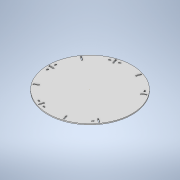
# Autodesk Inventor part: Base
Saved by Autodesk Inventor 2020 (Build 240168000, 168)
## iProperties
Created: 2020-07-30
Part Number: Base
Material: Generic
Document SubType Name: Modeling
Designer: Dan Wikman
Density: 1 g/cm^3
Appearance: Default
Author: Dan Wikman
Autodesk Inventor part; units mm, degrees
ref_plane "YZ Plane" through (0, 0, 0) normal (1, 0, 0) x (0, 1, 0)
ref_plane "XZ Plane" through (0, 0, 0) normal (0, 1, 0) x (-1, 0, 0)
ref_plane "XY Plane" through (0, 0, 0) normal (0, 0, 1) x (1, 0, 0)
sketch "Sketch1" plane through (0, 0, 0) normal (0, 1, 0) x (-1, 0, 0)
  circle A0 centre (0, 0) radius 300
  line L0 (290, 3.75) -> (260, 3.75)
  line L1 (260, -3.75) -> (290, -3.75)
  arc A1 (291.75, 2) -> (290, 3.75) centre (290, 2) ccw
  arc A2 (290, -3.75) -> (291.75, -2) centre (290, -2) ccw
  arc A3 (258.25, -2) -> (260, -3.75) centre (260, -2) ccw
  arc A4 (260, 3.75) -> (258.25, 2) centre (260, 2) ccw
  line L2 (258.25, 2) -> (258.25, -2)
  line L3 (291.75, -2) -> (291.75, 2)
  line L4 (306.241, 0) -> (300, 0)
  line L5 (300, 0) -> (281.7438, 0)
  line L6 (232.4107, 173.4915) -> (208.1402, 155.858)
  arc A5 (234.8551, 173.1044) -> (232.4107, 173.4915) centre (233.4394, 172.0758) ccw
  line L7 (237.2063, 169.8683) -> (234.8551, 173.1044)
  line L8 (212.5486, 149.7904) -> (236.8191, 167.4239)
  arc A6 (236.8191, 167.4239) -> (237.2063, 169.8683) centre (235.7905, 168.8397) ccw
  arc A7 (208.1402, 155.858) -> (207.7531, 153.4136) centre (209.1688, 154.4422) ccw
  line L9 (207.7531, 153.4136) -> (210.1042, 150.1775)
  arc A8 (210.1042, 150.1775) -> (212.5486, 149.7904) centre (211.52, 151.2061) ccw
  line L10 (86.0485, 276.9652) -> (76.778, 248.4335)
  arc A9 (88.2536, 278.0888) -> (86.0485, 276.9652) centre (87.7128, 276.4244) ccw
  line L11 (92.0578, 276.8527) -> (88.2536, 278.0888)
  line L12 (83.9109, 246.1159) -> (93.1814, 274.6476)
  arc A10 (93.1814, 274.6476) -> (92.0578, 276.8527) centre (91.517, 275.1884) ccw
  arc A11 (76.778, 248.4335) -> (77.9015, 246.2284) centre (78.4423, 247.8927) ccw
  line L13 (77.9015, 246.2284) -> (81.7058, 244.9923)
  arc A12 (81.7058, 244.9923) -> (83.9109, 246.1159) centre (82.2465, 246.6567) ccw
  line L14 (-93.1814, 274.6476) -> (-83.9109, 246.1159)
  arc A13 (-92.0578, 276.8527) -> (-93.1814, 274.6476) centre (-91.517, 275.1884) ccw
  line L15 (-88.2536, 278.0888) -> (-92.0578, 276.8527)
  line L16 (-76.778, 248.4335) -> (-86.0485, 276.9652)
  arc A14 (-86.0485, 276.9652) -> (-88.2536, 278.0888) centre (-87.7128, 276.4244) ccw
  arc A15 (-83.9109, 246.1159) -> (-81.7058, 244.9923) centre (-82.2465, 246.6567) ccw
  line L17 (-81.7058, 244.9923) -> (-77.9015, 246.2284)
  arc A16 (-77.9015, 246.2284) -> (-76.778, 248.4335) centre (-78.4423, 247.8927) ccw
  line L18 (-236.8191, 167.4239) -> (-212.5486, 149.7904)
  arc A17 (-237.2063, 169.8683) -> (-236.8191, 167.4239) centre (-235.7905, 168.8397) ccw
  line L19 (-234.8551, 173.1044) -> (-237.2063, 169.8683)
  line L20 (-208.1402, 155.858) -> (-232.4107, 173.4915)
  arc A18 (-232.4107, 173.4915) -> (-234.8551, 173.1044) centre (-233.4394, 172.0758) ccw
  arc A19 (-212.5486, 149.7904) -> (-210.1042, 150.1775) centre (-211.52, 151.2061) ccw
  line L21 (-210.1042, 150.1775) -> (-207.7531, 153.4136)
  arc A20 (-207.7531, 153.4136) -> (-208.1402, 155.858) centre (-209.1688, 154.4422) ccw
  line L22 (-232.4107, -173.4915) -> (-208.1402, -155.858)
  arc A21 (-234.8551, -173.1044) -> (-232.4107, -173.4915) centre (-233.4394, -172.0758) ccw
  line L23 (-237.2063, -169.8683) -> (-234.8551, -173.1044)
  line L24 (-212.5486, -149.7904) -> (-236.8191, -167.4239)
  arc A22 (-236.8191, -167.4239) -> (-237.2063, -169.8683) centre (-235.7905, -168.8397) ccw
  arc A23 (-208.1402, -155.858) -> (-207.7531, -153.4136) centre (-209.1688, -154.4422) ccw
  line L25 (-207.7531, -153.4136) -> (-210.1042, -150.1775)
  arc A24 (-210.1042, -150.1775) -> (-212.5486, -149.7904) centre (-211.52, -151.2061) ccw
  line L26 (-86.0485, -276.9652) -> (-76.778, -248.4335)
  arc A25 (-88.2536, -278.0888) -> (-86.0485, -276.9652) centre (-87.7128, -276.4244) ccw
  line L27 (-92.0578, -276.8527) -> (-88.2536, -278.0888)
  line L28 (-83.9109, -246.1159) -> (-93.1814, -274.6476)
  arc A26 (-93.1814, -274.6476) -> (-92.0578, -276.8527) centre (-91.517, -275.1884) ccw
  arc A27 (-76.778, -248.4335) -> (-77.9015, -246.2284) centre (-78.4423, -247.8927) ccw
  line L29 (-77.9015, -246.2284) -> (-81.7058, -244.9923)
  arc A28 (-81.7058, -244.9923) -> (-83.9109, -246.1159) centre (-82.2465, -246.6567) ccw
  line L30 (93.1814, -274.6476) -> (83.9109, -246.1159)
  arc A29 (92.0578, -276.8527) -> (93.1814, -274.6476) centre (91.517, -275.1884) ccw
  line L31 (88.2536, -278.0888) -> (92.0578, -276.8527)
  line L32 (76.778, -248.4335) -> (86.0485, -276.9652)
  arc A30 (86.0485, -276.9652) -> (88.2536, -278.0888) centre (87.7128, -276.4244) ccw
  arc A31 (83.9109, -246.1159) -> (81.7058, -244.9923) centre (82.2465, -246.6567) ccw
  line L33 (81.7058, -244.9923) -> (77.9015, -246.2284)
  arc A32 (77.9015, -246.2284) -> (76.778, -248.4335) centre (78.4423, -247.8927) ccw
  line L34 (236.8191, -167.4239) -> (212.5486, -149.7904)
  arc A33 (237.2063, -169.8683) -> (236.8191, -167.4239) centre (235.7905, -168.8397) ccw
  line L35 (234.8551, -173.1044) -> (237.2063, -169.8683)
  line L36 (208.1402, -155.858) -> (232.4107, -173.4915)
  arc A34 (232.4107, -173.4915) -> (234.8551, -173.1044) centre (233.4394, -172.0758) ccw
  arc A35 (212.5486, -149.7904) -> (210.1042, -150.1775) centre (211.52, -151.2061) ccw
  line L37 (210.1042, -150.1775) -> (207.7531, -153.4136)
  arc A36 (207.7531, -153.4136) -> (208.1402, -155.858) centre (209.1688, -154.4422) ccw
  point P0 (227.9355, 165.6049)
  point P1 (87.0636, 267.9543)
  point P2 (-87.0636, 267.9543)
  point P3 (-227.9355, 165.6049)
  point P4 (-227.9355, -165.6049)
  point P5 (-87.0636, -267.9543)
  point P6 (87.0636, -267.9543)
  point P7 (227.9355, -165.6049)
  dimension "d36" = 600
  dimension "d3" = 7.5
  dimension "d6" = 30
  dimension "d7" = 3.5
  dimension "d8" = 3.5
  dimension "d26" = 8.25
  dimension "d27" = 33.5
  dimension "d28" = 7.5
  constraints: 76 end point, 72 point on circle, 36 centre point, 4 tangent, 3 horizontal, 1 horizontal alignment, 1 parallel, 3 other
  measures "d3" distance between parallel lines of L1 L0
  measures "d6" distance of L1.start L1.end
  measures "d7" diameter of A1
  measures "d8" diameter of A2
  measures "d26" distance from line of L4.end L3
  measures "d27" distance between parallel lines of L2 L3
  measures "d28" diameter of L1 L5
extrude "Extrusion1" add sketch "Sketch1" along normal blind 7
sketch "Sketch2" plane through (0, 7, 0) normal (0, 1, 0) x (1, 0, 0)
  circle A0 centre (0, 0) radius 300 projected
  arc A1 (-260, -3.75) -> (-258.25, -2) centre (-260, -2) ccw projected
  line L0 (-260, -3.75) -> (-290, -3.75) projected
  arc A2 (-291.75, -2) -> (-290, -3.75) centre (-290, -2) ccw projected
  line L1 (-291.75, -2) -> (-291.75, 2) projected
  arc A3 (-290, 3.75) -> (-291.75, 2) centre (-290, 2) ccw projected
  line L2 (-290, 3.75) -> (-260, 3.75) projected
  arc A4 (-258.25, 2) -> (-260, 3.75) centre (-260, 2) ccw projected
  line L3 (-258.25, 2) -> (-258.25, -2) projected
  line L4 (-277, 22) -> (-273, 22)
  line L5 (-271.25, 23.75) -> (-271.25, 33.75)
  line L6 (-273, 35.5) -> (-277, 35.5)
  line L7 (-278.75, 33.75) -> (-278.75, 23.75)
  arc A5 (-273, 22) -> (-271.25, 23.75) centre (-273, 23.75) ccw
  arc A6 (-278.75, 23.75) -> (-277, 22) centre (-277, 23.75) ccw
  arc A7 (-277, 35.5) -> (-278.75, 33.75) centre (-277, 33.75) ccw
  arc A8 (-271.25, 33.75) -> (-273, 35.5) centre (-273, 33.75) ccw
  line L8 (-300, 0) -> (0, 0)
  line L9 (-277, -22) -> (-273, -22)
  line L10 (-271.25, -23.75) -> (-271.25, -33.75)
  line L11 (-273, -35.5) -> (-277, -35.5)
  line L12 (-278.75, -33.75) -> (-278.75, -23.75)
  arc A9 (-271.25, -23.75) -> (-273, -22) centre (-273, -23.75) ccw
  arc A10 (-277, -22) -> (-278.75, -23.75) centre (-277, -23.75) ccw
  arc A11 (-278.75, -33.75) -> (-277, -35.5) centre (-277, -33.75) ccw
  arc A12 (-273, -35.5) -> (-271.25, -33.75) centre (-273, -33.75) ccw
  arc A13 (-105.2849, -252.8401) -> (-106.4085, -250.6349) centre (-106.9492, -252.2993) ccw
  arc A14 (-119.3602, -252.4726) -> (-118.2366, -254.6777) centre (-117.6959, -253.0133) ccw
  line L13 (-118.1241, -248.6683) -> (-119.3602, -252.4726)
  arc A15 (-115.919, -247.5448) -> (-118.1241, -248.6683) centre (-116.4598, -249.2091) ccw
  line L14 (-106.4085, -250.6349) -> (-115.919, -247.5448)
  line L15 (-106.521, -256.6443) -> (-105.2849, -252.8401)
  arc A16 (-108.7261, -257.7679) -> (-106.521, -256.6443) centre (-108.1853, -256.1035) ccw
  line L16 (-118.2366, -254.6777) -> (-108.7261, -257.7679)
  line L17 (-64.6745, -270.241) -> (-63.4384, -266.4368)
  arc A17 (-61.2333, -265.3132) -> (-63.4384, -266.4368) centre (-61.774, -266.9776) ccw
  arc A18 (-64.6745, -270.241) -> (-63.5509, -272.4462) centre (-63.0101, -270.7818) ccw
  line L18 (-61.2333, -265.3132) -> (-51.7227, -268.4034)
  line L19 (-54.0403, -275.5363) -> (-63.5509, -272.4462)
  arc A19 (-50.5991, -270.6085) -> (-51.7227, -268.4034) centre (-52.2635, -270.0678) ccw
  line L20 (-50.5991, -270.6085) -> (-51.8352, -274.4128)
  arc A20 (-54.0403, -275.5363) -> (-51.8352, -274.4128) centre (-53.4996, -273.872) ccw
  arc A21 (207.9304, -178.2637) -> (205.486, -178.6509) centre (206.9017, -179.6795) ccw
  arc A22 (203.2313, -191.5366) -> (205.6757, -191.1495) centre (204.26, -190.1208) ccw
  line L21 (199.9953, -189.1855) -> (203.2313, -191.5366)
  arc A23 (199.6081, -186.7411) -> (199.9953, -189.1855) centre (201.0239, -187.7697) ccw
  line L22 (205.486, -178.6509) -> (199.6081, -186.7411)
  line L23 (211.1664, -180.6149) -> (207.9304, -178.2637)
  arc A24 (211.5536, -183.0593) -> (211.1664, -180.6149) centre (210.1378, -182.0307) ccw
  line L24 (205.6757, -191.1495) -> (211.5536, -183.0593)
  line L25 (211.1664, 180.6149) -> (207.9304, 178.2637)
  arc A25 (205.486, 178.6509) -> (207.9304, 178.2637) centre (206.9017, 179.6795) ccw
  arc A26 (211.1664, 180.6149) -> (211.5536, 183.0593) centre (210.1378, 182.0307) ccw
  line L26 (205.486, 178.6509) -> (199.6081, 186.7411)
  line L27 (205.6757, 191.1495) -> (211.5536, 183.0593)
  arc A27 (199.9953, 189.1855) -> (199.6081, 186.7411) centre (201.0239, 187.7697) ccw
  line L28 (199.9953, 189.1855) -> (203.2313, 191.5366)
  arc A28 (205.6757, 191.1495) -> (203.2313, 191.5366) centre (204.26, 190.1208) ccw
  arc A29 (-63.4384, 266.4368) -> (-61.2333, 265.3132) centre (-61.774, 266.9776) ccw
  arc A30 (-51.8352, 274.4128) -> (-54.0403, 275.5363) centre (-53.4996, 273.872) ccw
  line L29 (-50.5991, 270.6085) -> (-51.8352, 274.4128)
  arc A31 (-51.7227, 268.4034) -> (-50.5991, 270.6085) centre (-52.2635, 270.0678) ccw
  line L30 (-61.2333, 265.3132) -> (-51.7227, 268.4034)
  line L31 (-64.6745, 270.241) -> (-63.4384, 266.4368)
  arc A32 (-63.5509, 272.4462) -> (-64.6745, 270.241) centre (-63.0101, 270.7818) ccw
  line L32 (-54.0403, 275.5363) -> (-63.5509, 272.4462)
  line L33 (-106.521, 256.6443) -> (-105.2849, 252.8401)
  arc A33 (-106.4085, 250.6349) -> (-105.2849, 252.8401) centre (-106.9492, 252.2993) ccw
  arc A34 (-106.521, 256.6443) -> (-108.7261, 257.7679) centre (-108.1853, 256.1035) ccw
  line L34 (-106.4085, 250.6349) -> (-115.919, 247.5448)
  line L35 (-118.2366, 254.6777) -> (-108.7261, 257.7679)
  arc A35 (-118.1241, 248.6683) -> (-115.919, 247.5448) centre (-116.4598, 249.2091) ccw
  line L36 (-118.1241, 248.6683) -> (-119.3602, 252.4726)
  arc A36 (-118.2366, 254.6777) -> (-119.3602, 252.4726) centre (-117.6959, 253.0133) ccw
  dimension "d14" = 7.5
  dimension "d16" = 13
  dimension "d17" = 13
  dimension "d18" = 13.5
  dimension "d19" = 1.75
  dimension "d20" = 20
  constraints: 66 end point, 64 point on circle, 32 centre point, 12 symmetric about line, 8 tangent, 3 equal radius, 2 horizontal, 2 parallel, 1 perpendicular, 4 other
  measures "d14" distance between parallel lines of L5 L7
  measures "d16" distance between parallel lines of L3 L5
  measures "d17" distance between parallel lines of L1 L7
  measures "d18" distance between parallel lines of L6 L4
  measures "d19" radius of A5
  measures "d20" distance from line of L2 A6.centre
extrude "Extrusion2" cut sketch "Sketch2" against normal through all contours A6 L7 A7 L6 A8 L5 A5 L4 | L9 A9 L10 A12 L11 A11 L12 A10 | L15 A16 L16 A14 L13 A15 L14 A13 | L17 A17 L18 A19 L20 A20 L19 A18 | L23 A24 L24 A22 L21 A23 L22 A21 | L25 A25 L26 A27 L28 A28 L27 A26 | L31 A32 L32 A30 L29 A31 L30 A29 | L33 A33 L34 A35 L36 A36 L35 A34
body "Solid1"
